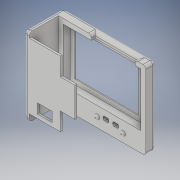
# Autodesk Inventor part: case top
Saved by Autodesk Inventor 2017 (Build 210142000, 142)
## iProperties
Created: 2016-12-04
Part Number: case top
Material: Generic
Document SubType Name: Modeling
Designer: radrajith
Density: 1 g/cm^3
Appearance: Default
Author: radrajith
Autodesk Inventor part; units mm, degrees
ref_plane "YZ Plane" through (0, 0, 0) normal (1, 0, 0) x (0, 1, 0)
ref_plane "XZ Plane" through (0, 0, 0) normal (0, 1, 0) x (-1, 0, 0)
ref_plane "XY Plane" through (0, 0, 0) normal (0, 0, 1) x (1, 0, 0)
sketch "Sketch1" plane through (0, 0, 0) normal (0, 0, 1) x (1, 0, 0)
  line L0 (0, 0) -> (95, 0)
  line L1 (95, 0) -> (95, 80)
  line L2 (95, 80) -> (0, 80)
  line L3 (0, 80) -> (0, 0)
  dimension "d0" = 95
  dimension "d1" = 80
  constraints: 8 end point, 2 parallel, 1 horizontal, 1 perpendicular
  measures "d0" distance of L2.end L1.end
  measures "d1" distance of L1.end L0.end
extrude "Extrusion1" add sketch "Sketch1" along normal blind 10
sketch "Sketch2" plane through (0, 0, 10) normal (0, 0, 1) x (1, 0, 0)
  line L0 (0, 0) -> (5, 0)
  line L1 (5, 0) -> (5, 80)
  line L2 (5, 80) -> (0, 80)
  line L3 (0, 80) -> (0, 0)
  dimension "d4" = 5
  dimension "d5" = 80
  constraints: 8 end point, 2 parallel, 1 horizontal, 1 perpendicular
  measures "d4" distance of L2.end L1.end
  measures "d5" distance of L1.end L0.end
extrude "Extrusion2" add sketch "Sketch2" along normal blind 30
sketch "Sketch3" plane through (5, 0, 10) normal (1, 0, 0) x (0, 0, -1)
  line L0 (-30, 80) -> (-30, 0) projected
  line L1 (-30, 7.5) -> (-28, 7.5)
  line L2 (-28, 7.5) -> (-28, 75)
  line L3 (-28, 75) -> (-30, 75)
  line L4 (-30, 75) -> (-30, 7.5)
  point P0 (10, 0)
  dimension "d8" = 2
  dimension "d9" = 67.5
  constraints: 8 end point, 2 parallel, 1 horizontal, 1 perpendicular, 1 point on line
  measures "d8" distance of L3.end L2.end
  measures "d9" distance of L2.end L1.end
extrude "Extrusion3" add sketch "Sketch3" along normal blind 47
sketch "Sketch4" plane through (52, 0, 10) normal (1, 0, 0) x (0, 0, -1)
  line L0 (-28, 75) -> (-28, 7.5) projected
  line L1 (-28, 75) -> (-30, 75)
  line L2 (-30, 75) -> (-30, 56.5)
  line L3 (-30, 56.5) -> (-28, 56.5)
  line L4 (-28, 56.5) -> (-28, 75)
  line L5 (-28, 7.5) -> (-30, 7.5)
  line L6 (-30, 7.5) -> (-30, 26)
  line L7 (-30, 26) -> (-28, 26)
  line L8 (-28, 26) -> (-28, 7.5)
  point P0 (10, 0)
  dimension "d12" = 2
  dimension "d13" = 18.5
  dimension "d14" = 2
  dimension "d15" = 18.5
  constraints: 16 end point, 4 parallel, 2 horizontal, 2 perpendicular
  measures "d12" distance of L3.end L2.end
  measures "d13" distance of L2.end L1.end
  measures "d14" distance of L6.end L7.end
  measures "d15" distance of L5.end L6.end
extrude "Extrusion4" cut sketch "Sketch4" against normal blind 15
sketch "Sketch5" plane through (0, 0, 40) normal (0, 0, 1) x (1, 0, 0)
  line L0 (28.5, 11.5) -> (13.5, 11.5)
  line L1 (13.5, 11.5) -> (13.5, 21.5)
  line L2 (13.5, 21.5) -> (28.5, 21.5)
  line L3 (28.5, 21.5) -> (28.5, 11.5)
  point P0 (0, 0)
  dimension "d18" = 15
  dimension "d19" = 10
  constraints: 8 end point, 2 parallel, 1 horizontal, 1 perpendicular
  measures "d18" distance of L1.end L2.end
  measures "d19" distance of L0.end L1.end
extrude "Extrusion5" cut sketch "Sketch5" against normal blind 2
sketch "Sketch6" plane through (0, 0, 0) normal (0, 0, -1) x (-1, 0, 0)
  line L0 (-80, 70) -> (-15, 70)
  line L1 (-15, 70) -> (-15, 25)
  line L2 (-15, 25) -> (-80, 25)
  line L3 (-80, 25) -> (-80, 70)
  line L4 (0, 80) -> (0, 0) projected
  line L5 (-95, 80) -> (0, 80) projected
  dimension "d22" = 65
  dimension "d23" = 45
  dimension "d24" = 15
  dimension "d25" = 10
  constraints: 8 end point, 2 parallel, 1 horizontal, 1 perpendicular
  measures "d22" distance of L1.end L2.end
  measures "d23" distance of L0.end L1.end
  measures "d24" distance between parallel lines of L4 L1
  measures "d25" distance between parallel lines of L5 L0
extrude "Extrusion6" cut sketch "Sketch6" against normal blind 10
sketch "Sketch7" plane through (0, 0, 0) normal (0, 0, -1) x (-1, 0, 0)
  point P0 (0, 0)
sketch "Sketch8" plane through (0, 0, 10) normal (0, 0, 1) x (1, 0, 0)
  line L0 (90, 20) -> (10, 20)
  line L1 (10, 20) -> (10, 75)
  line L2 (10, 75) -> (90, 75)
  line L3 (90, 75) -> (90, 20)
  point P0 (0, 0)
  dimension "d28" = 80
  dimension "d29" = 55
  constraints: 8 end point, 2 parallel, 1 horizontal, 1 perpendicular
  measures "d28" distance of L1.end L2.end
  measures "d29" distance of L0.end L1.end
extrude "Extrusion7" cut sketch "Sketch8" against normal blind 7
sketch "Sketch9" plane through (0, 0, 10) normal (0, 0, 1) x (1, 0, 0)
  circle A0 centre (45, 10) radius 2.5
  line L0 (0, 0) -> (95, 0) projected
  line L1 (5, 80) -> (5, 0) projected
  dimension "d32" = 5
  dimension "d36" = 10
  dimension "d41" = 40
  constraints: 1 centre point
  measures "d32" diameter of A0
  measures "d36" distance from line of L0 A0.centre
  measures "d41" distance from line of L1 A0.centre
extrude "Extrusion8" add sketch "Sketch9" along normal blind 2
fillet "Fillet1" radius 2 1 edges at (42.5, 10, 12)
sketch "Sketch10" plane through (0, 0, 10) normal (0, 0, 1) x (1, 0, 0)
  circle A0 centre (71.5, 8.5) radius 2.5
  point P0 (0, 0)
  dimension "d37" = 5
  constraints: 1 centre point
  measures "d37" diameter of A0
extrude "Extrusion9" add sketch "Sketch10" along normal blind 2
fillet "Fillet2" radius 2 1 edges at (69, 8.5, 12)
fillet "Fillet3" radius 3 1 edges at (95, 0, 5)
fillet "Fillet4" radius 3 3 edges at (46, 0, 0) (94.1213, 0.8787, 0) (95, 41.5, 0)
fillet "Fillet5" radius 3 3 edges at (0, 41.5, 0) (0, 0.8787, 0.8787) (0, 0, 21.5)
fillet "Fillet6" radius 3 5 edges at (47.5, 80, 0) (0.8787, 80, 0.8787) (0, 80, 21.5) (94.1213, 80, 0.8787) (95, 80, 6.5)
fillet "Fillet7" radius 3 5 edges at (0, 40, 40) (0.8787, 0.8787, 40) (4, 0, 40) (0.8787, 79.1213, 40) (4, 80, 40)
chamfer "Chamfer1" distance 2 angle 45 1 edges at (47.5, 25, 0)
chamfer "Chamfer2" distance 2 angle 45 1 edges at (15, 47.5, 0)
chamfer "Chamfer3" distance 2 angle 45 1 edges at (80, 47.5, 0)
sketch "Sketch11" plane through (0, 0, 0) normal (0, 0, -1) x (-1, 0, 0)
  line L0 (-65.5, 10) -> (-62.5, 10)
  line L1 (-61, 11.5) -> (-61, 12.5)
  line L2 (-62.5, 14) -> (-65.5, 14)
  line L3 (-67, 12.5) -> (-67, 11.5)
  line L4 (-55.5, 10) -> (-52.5, 10)
  line L5 (-51, 11.5) -> (-51, 12.5)
  line L6 (-52.5, 14) -> (-55.5, 14)
  line L7 (-57, 12.5) -> (-57, 11.5)
  arc A0 (-51, 12.5) -> (-52.5, 14) centre (-52.5, 12.5) ccw
  arc A1 (-52.5, 10) -> (-51, 11.5) centre (-52.5, 11.5) ccw
  arc A2 (-57, 11.5) -> (-55.5, 10) centre (-55.5, 11.5) ccw
  arc A3 (-55.5, 14) -> (-57, 12.5) centre (-55.5, 12.5) ccw
  arc A4 (-61, 12.5) -> (-62.5, 14) centre (-62.5, 12.5) ccw
  arc A5 (-62.5, 10) -> (-61, 11.5) centre (-62.5, 11.5) ccw
  arc A6 (-67, 11.5) -> (-65.5, 10) centre (-65.5, 11.5) ccw
  arc A7 (-65.5, 14) -> (-67, 12.5) centre (-65.5, 12.5) ccw
  point P0 (0, 0)
  point P1 (-67, 10)
  point P2 (-61, 14)
  point P3 (-61, 10)
  point P4 (-67, 14)
  point P5 (-57, 10)
  point P6 (-51, 14)
  point P7 (-51, 10)
  point P8 (-57, 14)
  dimension "d56" = 6
  dimension "d57" = 4
  dimension "d60" = 1.5
  constraints: 18 point on line, 16 end point, 16 point on circle, 16 tangent, 8 centre point, 7 equal radius, 4 parallel, 2 horizontal, 2 perpendicular
  measures "d56" distance of point (-67, 14) point (-61, 14)
  measures "d57" distance of point (-61, 14) point (-61, 10)
  measures "d60" radius of A0
extrude "Extrusion10" cut sketch "Sketch11" against normal blind 10
chamfer "Chamfer4" distance 2 angle 45 1 edges at (47.5, 70, 0)
sketch "Sketch12" plane through (0, 0, 10) normal (0, 0, 1) x (1, 0, 0)
  line L0 (92, 80) -> (5, 80) projected
  line L1 (10, 75) -> (90, 75) projected
  line L2 (38.911, 80) -> (83.911, 80)
  line L3 (83.911, 80) -> (83.911, 75)
  line L4 (83.911, 75) -> (38.911, 75)
  line L5 (38.911, 75) -> (38.911, 80)
  point P0 (0, 0)
  dimension "d64" = 45
  constraints: 8 end point, 2 parallel, 2 point on line, 1 horizontal, 1 perpendicular
  measures "d64" distance of L3.end L4.end
extrude "Extrusion11" cut sketch "Sketch12" against normal blind 4
fillet "Fillet8" radius 3 1 edges at (61.411, 80, 6)
fillet "Fillet9" radius 3 2 edges at (83.911, 80, 4.5003) (83.911, 80, 8)
fillet "Fillet10" radius 3 2 edges at (38.911, 80, 4.5003) (38.911, 80, 8)
body "Solid1"
